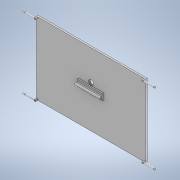
# Autodesk Inventor part: Bandeja
Saved by Autodesk Inventor 2021 (Build 250183000, 183)
## iProperties
Created: 2021-04-19
Part Number: Bandeja
Material: Genérico
Document SubType Name: Modeling
Designer: carlo
Density: 1 g/cm^3
Appearance: Valor por defecto
Author: carlo
Autodesk Inventor part; units mm, degrees
ref_plane "YZ Plane" through (0, 0, 0) normal (1, 0, 0) x (0, 1, 0)
ref_plane "XZ Plane" through (0, 0, 0) normal (0, 1, 0) x (-1, 0, 0)
ref_plane "XY Plane" through (0, 0, 0) normal (0, 0, 1) x (1, 0, 0)
sketch "Boceto1" plane through (0, 0, 0) normal (0, 0, 1) x (1, 0, 0)
  line L0 (-215, 142.5) -> (215, 142.5)
  line L1 (215, 142.5) -> (215, -142.5)
  line L2 (215, -142.5) -> (-215, -142.5)
  line L3 (-215, -142.5) -> (-215, 142.5)
  line L4 (-215, 142.5) -> (215, -142.5) construction
  line L5 (215, 142.5) -> (-215, -142.5) construction
  point P0 (0, 0)
  dimension "d0" = 430
  dimension "d1" = 285
  constraints: 12 end point, 2 midpoint, 2 parallel, 1 horizontal, 1 perpendicular
  measures "d0" distance of L1.end L2.end
  measures "d1" distance of L0.end L1.end
extrude "Extrusión1" add sketch "Boceto1" along normal blind 3
sketch "Boceto2" plane through (0, 0, 3) normal (0, 0, 1) x (1, 0, 0)
  line L0 (-50, -12.5) -> (50, -12.5)
  line L1 (50, -12.5) -> (50, 12.5)
  line L2 (50, 12.5) -> (-50, 12.5)
  line L3 (-50, 12.5) -> (-50, -12.5)
  line L4 (-50, -12.5) -> (50, 12.5) construction
  line L5 (50, -12.5) -> (-50, 12.5) construction
  point P0 (0, 0)
  dimension "d4" = 100
  dimension "d5" = 25
  constraints: 12 end point, 2 midpoint, 2 parallel, 1 horizontal, 1 perpendicular
  measures "d4" distance of L2.end L1.end
  measures "d5" distance of L1.end L0.end
extrude "Extrusión2" add sketch "Boceto2" along normal blind 5
sketch "Boceto3" plane through (50, -12.5, 3) normal (1, 0, 0) x (0, 0, -1)
  line L0 (-5, 0) -> (-5, 12.5)
  arc A0 (-10, 17.5) -> (-10, 7.5) centre (-10, 12.5) ccw
  circle A1 centre (-10, 12.5) radius 2.5
  line L1 (-5, 0) -> (-5, 25) projected
  line L2 (-10, 7.5) -> (-5, 7.5)
  line L3 (-5, 7.5) -> (-5, 17.5)
  line L4 (-5, 17.5) -> (-10, 17.5)
  point P0 (3, 12.5)
  dimension "d10" = 5
  constraints: 8 end point, 2 centre point, 2 point on circle, 1 coincident, 1 horizontal, 1 midpoint, 1 parallel, 1 perpendicular, 1 point on line
  measures "d10" diameter of A1
extrude "Extrusión3" add sketch "Boceto3" against normal blind 100
sketch "Boceto13" plane through (0, 0, 3) normal (0, 0, 1) x (1, 0, 0)
  line L0 (215, 142.5) -> (-215, 142.5) projected
  line L1 (-215, 142.5) -> (-210, 142.5)
  line L2 (-210, 142.5) -> (-210, 137.5)
  line L3 (-210, 137.5) -> (-215, 137.5)
  line L4 (-215, 137.5) -> (-215, 142.5)
  line L5 (215, -142.5) -> (215, 142.5) projected
  line L6 (215, 142.5) -> (210, 142.5)
  line L7 (210, 142.5) -> (210, 137.5)
  line L8 (210, 137.5) -> (215, 137.5)
  line L9 (215, 137.5) -> (215, 142.5)
  line L10 (-215, -142.5) -> (215, -142.5) projected
  line L11 (215, -142.5) -> (210, -142.5)
  line L12 (210, -142.5) -> (210, -137.5)
  line L13 (210, -137.5) -> (215, -137.5)
  line L14 (215, -137.5) -> (215, -142.5)
  line L15 (-215, -142.5) -> (-210, -142.5)
  line L16 (-210, -142.5) -> (-210, -137.5)
  line L17 (-210, -137.5) -> (-215, -137.5)
  line L18 (-215, -137.5) -> (-215, -142.5)
  point P0 (0, 0)
  dimension "d39" = 5
  dimension "d40" = 5
  dimension "d41" = 5
  dimension "d42" = 5
  dimension "d43" = 5
  dimension "d44" = 5
  dimension "d45" = 5
  dimension "d46" = 5
  constraints: 32 end point, 8 parallel, 4 horizontal, 4 perpendicular
  measures "d39" distance of L2.end L3.end
  measures "d40" distance of L1.end L2.end
  measures "d41" distance of L8.end L7.end
  measures "d42" distance of L7.end L6.end
  measures "d43" distance of L12.end L13.end
  measures "d44" distance of L11.end L12.end
  measures "d45" distance of L17.end L16.end
  measures "d46" distance of L16.end L15.end
extrude "Extrusión10" add sketch "Boceto13" along normal blind 10
sketch "Boceto16" plane through (-215, -142.5, 0) normal (-1, 0, 0) x (0, 0, 1)
  line L0 (13, 5) -> (13, 0) projected
  circle A0 centre (10.5, 2.5) radius 2.5
  line L1 (13, 285) -> (13, 280) projected
  circle A1 centre (10.5, 282.5) radius 2.5
  point P0 (0, 142.5)
  constraints: 2 centre point
extrude "Extrusión13" add sketch "Boceto16" along normal blind 45
sketch "Boceto17" plane through (215, -142.5, 0) normal (1, 0, 0) x (0, 0, -1)
  line L0 (-13, 280) -> (-13, 285) projected
  circle A0 centre (-10.5, 282.5) radius 2.5
  line L1 (-13, 0) -> (-13, 5) projected
  circle A1 centre (-10.5, 2.5) radius 2.5
  point P0 (0, 142.5)
  constraints: 2 centre point
extrude "Extrusión14" add sketch "Boceto17" along normal blind 45
ref_plane "Plano de trabajo3" through (-215, 140, 0) normal (0, 1, 0) x (1, 0, 0)
sketch "Boceto18" plane through (-215, 140, 0) normal (0, 1, 0) x (1, 0, 0)
  line L0 (475, -13) -> (475, -8) projected
  line L1 (475, -10.5) -> (470.5, -10.5)
  line L2 (470.5, -10.5) -> (470.5, -13)
  line L3 (430, -13) -> (475, -13) projected
  line L4 (470, -13.5) -> (471, -13.5)
  line L5 (471, -13.5) -> (471, -12.5)
  line L6 (471, -12.5) -> (470, -12.5)
  line L7 (470, -12.5) -> (470, -13.5)
  line L8 (470, -13.5) -> (471, -12.5) construction
  line L9 (471, -13.5) -> (470, -12.5) construction
  line L10 (-45, -8) -> (-45, -13) projected
  line L11 (-45, -10.5) -> (-38.08, -10.5)
  line L12 (-38.08, -10.5) -> (-38.08, -13)
  line L13 (0, -13) -> (-45, -13) projected
  line L14 (-38.58, -13.5) -> (-37.58, -13.5)
  line L15 (-37.58, -13.5) -> (-37.58, -12.5)
  line L16 (-37.58, -12.5) -> (-38.58, -12.5)
  line L17 (-38.58, -12.5) -> (-38.58, -13.5)
  line L18 (-38.58, -13.5) -> (-37.58, -12.5) construction
  line L19 (-37.58, -13.5) -> (-38.58, -12.5) construction
  point P0 (215, 0)
  point P1 (470, -13)
  point P2 (471, -13)
  dimension "d68" = 4.5
  dimension "d69" = 1
  dimension "d70" = 1
  dimension "d72" = 6.92
  dimension "d73" = 1
  dimension "d74" = 1
  constraints: 32 end point, 6 midpoint, 4 horizontal, 4 parallel, 3 perpendicular, 2 point on line, 1 vertical
  measures "d68" distance of L1.start L1.end
  measures "d69" distance of L6.end L5.end
  measures "d70" distance of L5.end L4.end
  measures "d72" distance of L11.start L11.end
  measures "d73" distance of L16.end L15.end
  measures "d74" distance of L15.end L14.end
revolve "Revolución1" cut sketch "Boceto18" angle 360 about axis through (260, 140, 10.5) along (-1, 0, 0) contours L3 L2 L6 L5 | L3 L7 L6 L2 | L17 L16 L12 L13 | L13 L15 L14 L17 | L16 L15 L13 L12
ref_plane "Plano de trabajo4" through (210, -140, 3) normal (0, 1, 0) x (1, 0, 0)
sketch "Boceto19" plane through (210, -140, 3) normal (0, 1, 0) x (1, 0, 0)
  line L0 (50, -10) -> (50, -5) projected
  line L1 (50, -7.5) -> (45.5, -7.5)
  line L2 (45.5, -7.5) -> (45.5, -10)
  line L3 (5, -10) -> (50, -10) projected
  line L4 (46, -10.5) -> (45, -10.5)
  line L5 (45, -10.5) -> (45, -9.5)
  line L6 (45, -9.5) -> (46, -9.5)
  line L7 (46, -9.5) -> (46, -10.5)
  line L8 (46, -10.5) -> (45, -9.5) construction
  line L9 (45, -10.5) -> (46, -9.5) construction
  line L10 (-470, -5) -> (-470, -10) projected
  line L11 (-470, -7.5) -> (-463.08, -7.5)
  line L12 (-463.08, -7.5) -> (-463.08, -10)
  line L13 (-462.58, -10) -> (-462.58, -5) projected
  line L14 (-463.58, -10.5) -> (-462.58, -10.5)
  line L15 (-462.58, -10.5) -> (-462.58, -9.5)
  line L16 (-462.58, -9.5) -> (-463.58, -9.5)
  line L17 (-463.58, -9.5) -> (-463.58, -10.5)
  line L18 (-463.58, -10.5) -> (-462.58, -9.5) construction
  line L19 (-462.58, -10.5) -> (-463.58, -9.5) construction
  point P0 (-210, 3)
  dimension "d76" = 4.5
  dimension "d77" = 1
  dimension "d78" = 1
  dimension "d79" = 6.92
  dimension "d80" = 1
  constraints: 32 end point, 6 midpoint, 4 horizontal, 4 parallel, 3 perpendicular, 2 point on line, 1 vertical
  measures "d76" distance of L1.start L1.end
  measures "d77" distance of L5.end L6.end
  measures "d78" distance of L4.end L5.end
  measures "d79" distance of L11.start L11.end
  measures "d80" distance of L15.end L14.end
revolve "Revolución2" cut sketch "Boceto19" angle 360 about axis through (260, -140, 10.5) along (-1, 0, 0) contours L7 L4 L5 L3 | L3 L2 L6 L7 | L3 L5 L6 L2 | L15 L14 L17 L16 L13
sketch "Sketch20" plane through (0, 0, 0) normal (0, 0, -1) x (-1, 0, 0)
  line L0 (215, 142.5) -> (215, -142.5) projected
  line L1 (215, -142.5) -> (-215, -142.5) projected
  line L2 (-215, 142.5) -> (215, 142.5) projected
  line L3 (-215, -142.5) -> (-215, 142.5) projected
  point P0 (0, 0)
extrude "Extrusion15" add sketch "Sketch20" along normal blind 3
sketch "Sketch22" plane through (0, 0, -3) normal (0, 0, -1) x (-1, 0, 0)
  line L0 (0, 0) -> (0, 23) construction
  circle A0 centre (0, 23) radius 9.5
  dimension "d84" = 23
  dimension "d85" = 19
  constraints: 2 end point, 1 centre point, 1 coincident, 1 vertical
  measures "d84" distance of L0.start L0.end
  measures "d85" diameter of A0
extrude "Extrusion16" cut sketch "Sketch22" against normal blind 6
